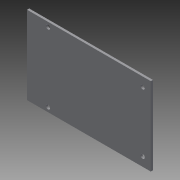
# Autodesk Inventor part: BBB固定板
Saved by Autodesk Inventor 2014 (Build 180170000, 170)
## iProperties
Created: 2013-09-12
Part Number: BBB固定板
Material: 一般
Document SubType Name: Modeling
Designer: koki
Density: 1 g/cm^3
Appearance: 既定
Author: koki
Autodesk Inventor part; units mm, degrees
ref_plane "YZ Plane" through (0, 0, 0) normal (1, 0, 0) x (0, 1, 0)
ref_plane "XZ Plane" through (0, 0, 0) normal (0, 1, 0) x (-1, 0, 0)
ref_plane "XY Plane" through (0, 0, 0) normal (0, 0, 1) x (1, 0, 0)
sketch "スケッチ1" plane through (0, 0, 0) normal (0, 1, 0) x (-1, 0, 0)
  line L0 (1.3839, 6.0339) -> (87.7439, 6.0339)
  line L1 (87.7439, 6.0339) -> (87.7439, -48.5761)
  line L2 (87.7439, -48.5761) -> (1.3839, -48.5761)
  line L3 (1.3839, -48.5761) -> (1.3839, 6.0339)
  point P0 (0, 0)
  point P1 (15.9889, 2.8589)
  point P2 (15.9889, -45.4011)
  point P3 (82.0289, -42.2261)
  point P4 (82.0289, -0.3161)
  dimension "d0" = 86.36
  dimension "d1" = 54.61
  dimension "d4" = 14.605
  dimension "d5" = 3.175
  dimension "d6" = 3.175
  dimension "d7" = 14.605
  dimension "d8" = 6.35
  dimension "d9" = 5.715
  dimension "d10" = 6.35
  dimension "d11" = 5.715
  constraints: 8 end point, 2 parallel, 1 horizontal, 1 perpendicular
  measures "d0" distance of L1.end L2.end
  measures "d1" distance of L0.end L1.end
  measures "d4" distance from line of L3 point (15.989, 2.859)
  measures "d5" distance from line of L0 point (15.989, 2.859)
  measures "d6" distance from line of L2 point (15.989, -45.401)
  measures "d7" distance from line of L3 point (15.989, -45.401)
  measures "d8" distance from line of L2 point (82.029, -42.226)
  measures "d9" distance from line of L1 point (82.029, -42.226)
  measures "d10" distance from line of L0 point (82.029, -0.316)
  measures "d11" distance from line of L1 point (82.029, -0.316)
extrude "押し出し1" add sketch "スケッチ1" along normal blind 1.5
sketch "スケッチ2" plane through (0, 1.5, 0) normal (0, 1, 0) x (1, 0, 0)
  line L0 (-1.3839, 48.5761) -> (-87.7439, 48.5761) projected
  line L1 (-87.7439, 48.5761) -> (-87.7439, -6.0339) projected
  line L2 (-87.7439, 48.5761) -> (-1.3839, 48.5761)
  line L3 (-1.3839, 48.5761) -> (-1.3839, -6.0339)
  line L4 (-1.3839, -6.0339) -> (-87.7439, -6.0339)
  line L5 (-87.7439, -6.0339) -> (-87.7439, 48.5761)
  point P0 (0, 0)
  point P1 (0, 0)
  point P2 (-73.1389, 45.4011)
  point P3 (-73.1389, -2.8589)
  point P4 (-7.0989, 0.3161)
  point P5 (-7.0989, 42.2261)
  dimension "d12" = 86.36
  dimension "d13" = 54.61
  dimension "d14" = 14.605
  dimension "d15" = 3.175
  dimension "d16" = 3.175
  dimension "d17" = 14.605
  dimension "d18" = 6.35
  dimension "d19" = 5.715
  dimension "d20" = 6.35
  dimension "d21" = 5.715
  dimension "d22" = 0
  dimension "d23" = 0
  constraints: 8 end point, 2 parallel, 1 horizontal, 1 perpendicular
  measures "d12" distance of L3.end L4.end
  measures "d13" distance of L2.end L3.end
  measures "d14" distance from line of L5 point (-73.139, 45.401)
  measures "d15" distance from line of L2 point (-73.139, 45.401)
  measures "d16" distance from line of L4 point (-73.139, -2.859)
  measures "d17" distance from line of L5 point (-73.139, -2.859)
  measures "d18" distance from line of L4 point (-7.099, 0.316)
  measures "d19" distance from line of L3 point (-7.099, 0.316)
  measures "d20" distance from line of L2 point (-7.099, 42.226)
  measures "d21" distance from line of L3 point (-7.099, 42.226)
  measures "d22" distance between parallel lines of L0 L2
  measures "d23" distance between parallel lines of L1 L5
hole "穴1" at (-7.0989, 1.5, -42.2261) at (-7.0989, 1.5, -0.3161) at (-73.1389, 1.5, 2.8589) at (-73.1389, 1.5, -45.4011) direction (0, -1, 0) diameter 3 end through all
